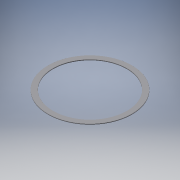
# Autodesk Inventor part: 鐵弗龍間隔環
Saved by Autodesk Inventor 2018 (Build 220112000, 112)
## iProperties
Created: 2021-09-16
Part Number: 鐵弗龍間隔環
Material: 一般
Document SubType Name: Modeling
Designer: user
Density: 1 g/cm^3
Appearance: 預設
Author: user
Autodesk Inventor part; units mm, degrees
ref_plane "YZ Plane" through (0, 0, 0) normal (1, 0, 0) x (0, 1, 0)
ref_plane "XZ Plane" through (0, 0, 0) normal (0, 1, 0) x (-1, 0, 0)
ref_plane "XY Plane" through (0, 0, 0) normal (0, 0, 1) x (1, 0, 0)
sketch "草圖1" plane through (0, 0, 0) normal (0, 0, 1) x (1, 0, 0)
  circle A0 centre (0, 0) radius 135
  circle A1 centre (0, 0) radius 153.85
  dimension "d0" = 270
  dimension "d1" = 18.85
  dimension "d2" = 307.7
  constraints: 2 centre point, 2 coincident
  measures "d0" diameter of A0
  measures "d1" radial gap between concentric circles of A1 A0
  measures "d2" diameter of A1
extrude "擠出1" add sketch "草圖1" along normal blind 3
chamfer "倒角1" distance 0.3 angle 45 2 edges at (-135, 0, 3) (-135, 0, 0)
chamfer "倒角2" distance 0.5 angle 45 2 edges at (-153.85, 0, 3) (-153.85, 0, 0)
